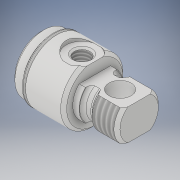
# Autodesk Inventor part: 02P0Y000_rear_head
Saved by Autodesk Inventor 2019 (Build 230136000, 136)
## iProperties
Created: 2023-02-02
Part Number: 02P0Y000_rear_head
Material: Generic
Catalog Web Link: www.cadenas.de
Description: Rear Head-Original Line - Standard Air Cylinders
Vendor: BIMBA
Document SubType Name: Modeling
Designer: psAdmin
Manufacturer: BIMBA
Mass: 2.8315 g
Surface Area: 17.5536 cm^2
Volume: 2.8315 cm^3
Density: 1 g/cm^3
Appearance: PSOLRGB-211-211-211
Category: PARTsolutions
Company: BIMBA
Title: 02P0Y000_rear_head
Author: Cadenas PARTsolutions
Comments: Original Line - Standard Air Cylinders
PSOL_IDENT_0: {$CADENAS_DATA/23d-libs/bimba/bimba_brand/bimba_imperial/bimba_full_line/original_line_cylinders/sta
PSOL_IDENT_1: ndard_air_cylinders/rear_head.prj},241 {VTYP=3D},{NB=02P0Y000_rear_head},{LINA=02P0Y000_rear_head},{
PSOL_IDENT_2: NN=Rear Head},{DATE=26.01.2023 11:43:55},{GEOMDATE=25.01.2022 07:32:02},{VERSION=},{LINEID=30},{WBVA
PSOL_IDENT_3: R=MNT,ACTING,DER,Q,T1,T2,T3,T4,TRIM,Y,K,MB,CUSH,FBON},{WBNUMERIC=TRIM,MB,CUSH}  {NB=02P0Y000_rear_he
PSOL_IDENT_4: ad},{LINA=02P0Y000_rear_head},{KT=DUMMY},{PN=02P0Y000},{BORE=0.56250},{BOREPN=02},{MNT=P},{MNTALG=''
PSOL_IDENT_5: , 'Front Nose' , 'P' , 'Rear Pivot' , 'DX' , 'Double End'},{ACTING=},{ACTINGALG= '' , 'Single Actin
PSOL_IDENT_6: g' },{DER=},{DERALG= '' , 'Standard' },{Q=},{T1=},{T2=},{T3=},{T4=},{TRIM=0},{Y=Y},{K=},{KALG= '', '
PSOL_IDENT_7: without K', 'K', 'with K' },{MB=0},{A1=0.9690},{A1N=0.5000},{A1P=0.9690},{A1B=0.0000},{A1S=0.0000},{
PSOL_IDENT_8: A2=0.157},{A2N=0.1570},{A3=0.0250},{D1=0.6150},{D1N=0.6095},{D1P=0.6150},{D1B=0.0000},{D2=0.5725},{C
PSOL_IDENT_9: 1=0.0300},{C2=0.0300},{NDM=0.1900},{TAB=UNF},{NDMDP=0.2000},{D3=0.1600},{A4=0.1830},{A5=0.4950},{D4=
PSOL_IDENT_10: 0.0000},{A6=0.0000},{A7=0.3750},{A8=0.0000},{D5=0.0000},{D6=0.1540},{A9=0.4400},{NDM2=0.4375},{TAB2=
PSOL_IDENT_11: UNF},{C11=0.0300},{C22=0.0000},{C33=0.0300},{C44=0.0300},{A10=0.3070},{A11=0.0000},{NDM3=0.1900},{ND
PSOL_IDENT_12: M3N=0.1900},{NDM3B=0.0000},{TAB3=UNF},{TAB3N=UNF},{TAB3B=-},{A12=0.406},{A12N=0.4060},{A12B=0.0000},
PSOL_IDENT_13: {A13=0.7810},{D7=0.1570},{D8=0.4355},{A14=0.0620},{A15=0.0775},{D9=0.3600},{R1=0.0315},{X1=0.0000},{
PSOL_IDENT_14: X2=0.0000},{CX=0.0000},{CC=0.0000},{CON=1},{S1=0.0000},{DB=0.0000},{X1B=0.0000},{X2B=0.0000},{A8B=0.
PSOL_IDENT_15: 0000},{A9B=0.0000},{MODEL=1},{NDM4=0.0000},{TAB4=-},{NDM4DP=0.0000},{BC=0.0000},{B1=0.0000},{B2=0.00
PSOL_IDENT_16: 00},{B3=0.0000},{ON=0},{ON2=1},{G1=0.0000},{G2=0.0000},{G3=0.0000},{G4=0.0000},{GD=0.0000},{G5=0.000
PSOL_IDENT_17: 0},{G6=0.0000},{RON=0},{H1=0.0000},{H2=0.0000},{H3=0.0000},{H4=0.0000},{H5=0.0000},{H6=0.0000},{F=0.
PSOL_IDENT_18: 0000},{PNUT=0.5940},{CUSH=0},{CC11=0.000},{CC111=0.0000},{CC22=0.0000},{CC33=0.0000},{CC44=0.0000},{
PSOL_IDENT_19: CC55=0.0000},{CD1=0.0000},{CD2=0.0000},{CD3=0.0000},{CNDM3=0.0000},{CTAB3=0.0000},{OLEN=0.7810},{OD=
PSOL_IDENT_20: 0.2185},{STDIS=0.6250},{STDIS1=0.1560},{BUSHCON=D-8597},{BUSHL=0.3120},{FBON=0},{LCD=0.0000}
NB: 02P0Y000_rear_head
NN: Rear Head
NT: Original Line - Standard Air Cylinders
NBSYN: $PN._rear_head
LINA: 02P0Y000_rear_head
CATALOG: Bimba Products
PN: 02P0Y000
BORE: 0.5625
BOREPN: 02
MNT: Rear Pivot
MNTALG: '' , 'Front Nose' , 'P' , 'Rear Pivot' , 'DX' , 'Double End'
ACTING: Single Acting
DER: Standard
Q: Without Side Ported Rear Head
T1: without T1
T2: without T2
T3: without T3
T4: without T4
TRIM: 0
Y: with Pivot Bushing
K: without K
MB: 0
A1N: 0.5
A1P: 0.969
A1B: 0
A1S: 0
A2N: 0.157
A3: 0.025
D1N: 0.6095
D1P: 0.615
D1B: 0
D2: 0.5725
C1: 0.03
C2: 0.03
TAB: UNF
NDMDP: 0.2
D3: 0.16
A4: 0.183
A5: 0.495
D4: 0
A6: 0
A7: 0.375
A8: 0
D5: 0
D6: 0.154
A9: 0.44
NDM2: 0.4375
TAB2: UNF
C11: 0.03
C22: 0
C33: 0.03
C44: 0.03
A10: 0.307
A11: 0
NDM3N: 0.19
NDM3B: 0
TAB3N: UNF
TAB3B: -
A12N: 0.406
A12B: 0
A13: 0.781
D7: 0.157
D8: 0.4355
A14: 0.062
A15: 0.0775
D9: 0.36
R1: 0.0315
X1: 0
X2: 0
CX: 0
CC: 0
S1: 0
DB: 0
X1B: 0
X2B: 0
A8B: 0
A9B: 0
NDM4: 0
TAB4: -
NDM4DP: 0
BC: 0
B1: 0
B2: 0
B3: 0
G1: 0
G2: 0
G3: 0
G4: 0
GD: 0
G5: 0
G6: 0
H2: 0
H3: 0
F: 0
CUSH: 0
CC111: 0
CC22: 0
CC33: 0
CC44: 0
CC55: 0
CD1: 0
CD2: 0
CD3: 0
CNDM3: 0
CTAB3: 0.0000
OD: 0.2185
STDIS1: 0.156
BUSHCON: D-8597
BUSHL: 0.312
FBON: 0
LCD: 0
SUPPLIER: BIMBA
ARTICLENO: 02P0Y000_rear_head
BOMINFO: 02P0Y000_rear_head
CREATOR: CADENAS GmbH
Autodesk Inventor part; units mm, degrees
sketch "Sketch_18" plane through (0, 0, 0) normal (0, 0, 1) x (1, 0, 0)
  line L0 (13.5128, 0) -> (0, 0)
  line L1 (0, 0) -> (0, 6.5088)
  line L2 (0, 6.5088) -> (0.762, 7.2708)
  line L3 (0.762, 7.2708) -> (2.7178, 7.2708)
  line L4 (2.7178, 7.2708) -> (3.3528, 6.6357)
  line L5 (3.3528, 6.6357) -> (3.9878, 6.6357)
  line L6 (3.9878, 6.6357) -> (3.9878, 7.8105)
  line L7 (3.9878, 7.8105) -> (12.7508, 7.8105)
  line L8 (12.7508, 7.8105) -> (13.5128, 7.0485)
  line L9 (13.5128, 7.0485) -> (13.5128, 0)
  line L10 (13.5128, 0) -> (0, 0)
  constraints: 22 end point
revolve "Revolution1" add sketch "Sketch_18" angle 360 about axis through (13.5128, 0, 0) along (1, 0, 0)
sketch "Sketch_15" plane through (0, 0, 0) normal (0, 0, 1) x (1, 0, 0)
  line L0 (24.6126, 0) -> (13.5128, 0)
  line L1 (13.5128, 0) -> (13.5128, 5.5309)
  line L2 (13.5128, 5.5309) -> (15.0876, 5.5309)
  line L3 (15.0876, 5.5309) -> (15.0876, 5.3721)
  arc A0 (15.0876, 5.3721) -> (15.8877, 4.572) centre (15.8877, 5.3721) ccw
  line L4 (15.8877, 4.572) -> (17.0561, 4.572)
  arc A1 (17.0561, 4.572) -> (17.559, 4.7498) centre (17.0561, 5.3721) ccw
  line L5 (17.559, 4.7498) -> (17.6219, 4.8006)
  line L6 (17.6219, 4.8006) -> (18.3775, 5.5563)
  line L7 (18.3775, 5.5563) -> (23.857, 5.5563)
  line L8 (23.857, 5.5563) -> (24.6126, 4.8006)
  line L9 (24.6126, 4.8006) -> (24.6126, 0)
  line L10 (24.6126, 0) -> (13.5128, 0)
  constraints: 22 end point, 4 point on circle, 2 centre point
revolve "Revolution2" add sketch "Sketch_15" angle 360 about axis through (24.6126, 0, 0) along (1, 0, 0)
thread "Thread1" size "7/16-20 UNF" class "2A" standard "ANSI Unified Screw Threads" full length
sketch "Sketch_70" plane through (24.6126, 0, 0) normal (1, 0, 0) x (0, 0, -1)
  line L0 (-31.242, -15.621) -> (31.242, -15.621)
  line L1 (31.242, -15.621) -> (31.242, 15.621)
  line L2 (31.242, 15.621) -> (-31.242, 15.621)
  line L3 (-31.242, 15.621) -> (-31.242, -15.621)
  line L4 (-15.621, -3.8989) -> (15.621, -3.8989)
  line L5 (15.621, -3.8989) -> (15.621, 3.8989)
  line L6 (15.621, 3.8989) -> (-15.621, 3.8989)
  line L7 (-15.621, 3.8989) -> (-15.621, -3.8989)
  constraints: 16 end point
extrude "Extrusion1" cut sketch "Sketch_70" against normal blind 11.0998
sketch "Sketch4" plane through (0, 0, 0) normal (-1, 0, 0) x (0, 0, 1)
  point P0 (0, 0)
hole "Hole1" at (0, 0, 0) direction (1, 0, 0) diameter 3.9116 depth 12.2936 tip angle 120
sketch "Sketch_45" plane through (0, 0, 0) normal (0, 0, 1) x (1, 0, 0)
  line L0 (10.3124, 6.7945) -> (10.3124, 7.8105)
  line L1 (10.3124, 7.8105) -> (14.2748, 7.8105)
  line L2 (14.2748, 7.8105) -> (14.2748, 6.7945)
  line L3 (14.2748, 6.7945) -> (10.3124, 6.7945)
  line L4 (10.3124, 6.7945) -> (10.3124, 7.8105)
  constraints: 10 end point
revolve "Revolution3" cut sketch "Sketch_45" angle 360 about axis through (10.3124, 6.7945, 0) along (0, -1, 0)
sketch "Sketch_46" plane through (0, 0, 0) normal (0, 0, 1) x (1, 0, 0)
  line L0 (10.3124, 0) -> (10.3124, 8.0645)
  line L1 (10.3124, 8.0645) -> (12.7254, 8.0645)
  line L2 (12.7254, 8.0645) -> (12.7254, 6.7945)
  line L3 (12.7254, 6.7945) -> (12.2961, 6.3652)
  line L4 (12.2961, 6.3652) -> (12.2961, 0)
  line L5 (12.2961, 0) -> (10.3124, 0)
  line L6 (10.3124, 0) -> (10.3124, 8.0645)
  constraints: 14 end point
revolve "Revolution4" cut sketch "Sketch_46" angle 360 about axis through (10.3124, 0, 0) along (0, -1, 0)
thread "Thread2" size "10-32 UNF" class "2B" standard "ANSI Unified Screw Threads" length 4.4094
sketch "Sketch_24" plane through (0, 0, 0) normal (0, 0, 1) x (1, 0, 0)
  line L0 (3.9878, 0) -> (3.3528, 0)
  line L1 (3.1602, 7.8105) -> (3.1602, 7.7263)
  line L2 (3.1602, 7.7263) -> (3.8708, 7.0158)
  arc A0 (3.8708, 6.8362) -> (3.8708, 7.0158) centre (3.781, 6.926) ccw
  line L3 (3.8708, 6.8362) -> (3.6703, 6.6357)
  line L4 (3.6703, 6.6357) -> (3.3528, 6.6357)
  line L5 (3.3528, 6.6357) -> (3.3528, 6.3817)
  line L6 (3.3528, 6.3817) -> (3.9878, 6.3817)
  line L7 (3.9878, 6.3817) -> (3.9878, 7.1861)
  line L8 (3.9878, 7.1861) -> (3.3634, 7.8105)
  line L9 (3.3634, 7.8105) -> (3.1602, 7.8105)
  constraints: 20 end point, 2 point on circle, 1 centre point
revolve "Revolution5" add sketch "Sketch_24" angle 360 about axis through (3.9878, 0, 0) along (1, 0, 0)
sketch "Sketch_43" plane through (0, 0, 0) normal (0, 1, 0) x (-1, 0, 0)
  circle A0 centre (-19.8374, 0) radius 2.775
  constraints: 1 centre point
extrude "Extrusion2" cut sketch "Sketch_43" along normal mid plane 11.6967
ref_plane "1_XY" through (15.0876, 0, 0) normal (1, 0, 0) x (0, 0, -1)
ref_plane "1_YZ" through (15.0876, 0, 0) normal (0, 0, -1) x (0, 1, 0)
ref_plane "1_ZX" through (15.0876, 0, 0) normal (0, 1, 0) x (1, 0, 0)
ref_plane "c1_XY" through (13.5128, 5.5309, 0) normal (0, 0, 1) x (1, 0, 0)
ref_plane "c1_YZ" through (13.5128, 5.5309, 0) normal (1, 0, 0) x (0, 1, 0)
ref_plane "c1_ZX" through (13.5128, 5.5309, 0) normal (0, 1, 0) x (0, 0, 1)
ref_plane "c2_XY" through (13.5128, -5.5309, 0) normal (0, 0, 1) x (1, 0, 0)
ref_plane "c2_YZ" through (13.5128, -5.5309, 0) normal (1, 0, 0) x (0, 1, 0)
ref_plane "c2_ZX" through (13.5128, -5.5309, 0) normal (0, 1, 0) x (0, 0, 1)
ref_plane "cc1_XY" through (13.5128, 0, 0) normal (0, 0, 1) x (1, 0, 0)
ref_plane "cc1_YZ" through (13.5128, 0, 0) normal (1, 0, 0) x (0, 1, 0)
ref_plane "cc1_ZX" through (13.5128, 0, 0) normal (0, 1, 0) x (0, 0, 1)
ref_plane "cc2_XY" through (15.0876, 0, 0) normal (0, 0, 1) x (1, 0, 0)
ref_plane "cc2_YZ" through (15.0876, 0, 0) normal (1, 0, 0) x (0, 1, 0)
ref_plane "cc2_ZX" through (15.0876, 0, 0) normal (0, 1, 0) x (0, 0, 1)
ref_plane "lovra1_XY" through (19.9644, 0, 0) normal (1, 0, 0) x (0, 0, -1)
ref_plane "lovra1_YZ" through (19.9644, 0, 0) normal (0, 0, -1) x (0, 1, 0)
ref_plane "lovra1_ZX" through (19.9644, 0, 0) normal (0, 1, 0) x (1, 0, 0)
ref_plane "lovra2_XY" through (19.9644, 6.2865, 0) normal (1, 0, 0) x (0, 0, -1)
ref_plane "lovra2_YZ" through (19.9644, 6.2865, 0) normal (0, 0, -1) x (0, 1, 0)
ref_plane "lovra2_ZX" through (19.9644, 6.2865, 0) normal (0, 1, 0) x (1, 0, 0)
ref_plane "lovra21_XY" through (0, 0, 5.2705) normal (1, 0, 0) x (0, 0, -1)
ref_plane "lovra21_YZ" through (0, 0, 5.2705) normal (0, 0, -1) x (0, 1, 0)
ref_plane "lovra21_ZX" through (0, 0, 5.2705) normal (0, 1, 0) x (1, 0, 0)
ref_plane "lovra22_XY" through (0, 0, -5.2705) normal (1, 0, 0) x (0, 0, -1)
ref_plane "lovra22_YZ" through (0, 0, -5.2705) normal (0, 0, -1) x (0, 1, 0)
ref_plane "lovra22_ZX" through (0, 0, -5.2705) normal (0, 1, 0) x (1, 0, 0)
ref_plane "lovra3_XY" through (19.9644, -6.2865, 0) normal (1, 0, 0) x (0, 0, -1)
ref_plane "lovra3_YZ" through (19.9644, -6.2865, 0) normal (0, 0, -1) x (0, 1, 0)
ref_plane "lovra3_ZX" through (19.9644, -6.2865, 0) normal (0, 1, 0) x (1, 0, 0)
ref_plane "olen_XY" through (19.8374, 0, 0) normal (1, 0, 0) x (0, 0, -1)
ref_plane "olen_YZ" through (19.8374, 0, 0) normal (0, 0, -1) x (0, 1, 0)
ref_plane "olen_ZX" through (19.8374, 0, 0) normal (0, 1, 0) x (1, 0, 0)
ref_plane "p1_XY" through (24.6126, 0, 3.9624) normal (1, 0, 0) x (0, 0, -1)
ref_plane "p1_YZ" through (24.6126, 0, 3.9624) normal (0, 0, -1) x (0, 1, 0)
ref_plane "p1_ZX" through (24.6126, 0, 3.9624) normal (0, 1, 0) x (1, 0, 0)
ref_plane "p2_XY" through (24.6126, 0, -3.9624) normal (1, 0, 0) x (0, 0, -1)
ref_plane "p2_YZ" through (24.6126, 0, -3.9624) normal (0, 0, -1) x (0, 1, 0)
ref_plane "p2_ZX" through (24.6126, 0, -3.9624) normal (0, 1, 0) x (1, 0, 0)
ref_plane "port_XY" through (10.3124, 0, 0) normal (0, 0, 1) x (1, 0, 0)
ref_plane "port_YZ" through (10.3124, 0, 0) normal (1, 0, 0) x (0, 1, 0)
ref_plane "port_ZX" through (10.3124, 0, 0) normal (0, 1, 0) x (0, 0, 1)
ref_plane "port2_XY" through (24.6126, 0, 0) normal (1, 0, 0) x (0, 0, -1)
ref_plane "port2_YZ" through (24.6126, 0, 0) normal (0, 0, -1) x (0, 1, 0)
ref_plane "port2_ZX" through (24.6126, 0, 0) normal (0, 1, 0) x (1, 0, 0)
ref_plane "thd1_XY" through (24.6126, 0, 5.5563) normal (1, 0, 0) x (0, 0, -1)
ref_plane "thd1_YZ" through (24.6126, 0, 5.5563) normal (0, 0, -1) x (0, 1, 0)
ref_plane "thd1_ZX" through (24.6126, 0, 5.5563) normal (0, 1, 0) x (1, 0, 0)
ref_plane "thd2_XY" through (24.6126, 0, -5.5563) normal (1, 0, 0) x (0, 0, -1)
ref_plane "thd2_YZ" through (24.6126, 0, -5.5563) normal (0, 0, -1) x (0, 1, 0)
ref_plane "thd2_ZX" through (24.6126, 0, -5.5563) normal (0, 1, 0) x (1, 0, 0)
ref_plane "to_mounting_bracket_XY" through (13.5128, 0, 0) normal (1, 0, 0) x (0, 0, -1)
ref_plane "to_mounting_bracket_YZ" through (13.5128, 0, 0) normal (0, 0, -1) x (0, 1, 0)
ref_plane "to_mounting_bracket_ZX" through (13.5128, 0, 0) normal (0, 1, 0) x (1, 0, 0)
ref_plane "to_nut_XY" through (15.0876, 0, 0) normal (1, 0, 0) x (0, 0, -1)
ref_plane "to_nut_YZ" through (15.0876, 0, 0) normal (0, 0, -1) x (0, 1, 0)
ref_plane "to_nut_ZX" through (15.0876, 0, 0) normal (0, 1, 0) x (1, 0, 0)
ref_plane "to_pin_XY" through (19.8374, 0, 0) normal (0, 1, 0) x (1, 0, 0)
ref_plane "to_pin_YZ" through (19.8374, 0, 0) normal (1, 0, 0) x (0, 0, -1)
ref_plane "to_pin_ZX" through (19.8374, 0, 0) normal (0, 0, -1) x (0, 1, 0)
ref_plane "to_pin_1_XY" through (19.8374, 0, 0) normal (0, 0, 1) x (1, 0, 0)
ref_plane "to_pin_1_YZ" through (19.8374, 0, 0) normal (1, 0, 0) x (0, 1, 0)
ref_plane "to_pin_1_ZX" through (19.8374, 0, 0) normal (0, 1, 0) x (0, 0, 1)
ref_plane "to_pin_r_XY" through (19.8374, 0, 0) normal (0, 0, 1) x (1, 0, 0)
ref_plane "to_pin_r_YZ" through (19.8374, 0, 0) normal (1, 0, 0) x (0, 1, 0)
ref_plane "to_pin_r_ZX" through (19.8374, 0, 0) normal (0, 1, 0) x (0, 0, 1)
ref_plane "to_screw_XY" through (10.3124, 0, 0) normal (0, 1, 0) x (1, 0, 0)
ref_plane "to_screw_YZ" through (10.3124, 0, 0) normal (1, 0, 0) x (0, 0, -1)
ref_plane "to_screw_ZX" through (10.3124, 0, 0) normal (0, 0, -1) x (0, 1, 0)
ref_plane "to_tube_XY" through (3.3528, 0, 0) normal (1, 0, 0) x (0, 0, -1)
ref_plane "to_tube_YZ" through (3.3528, 0, 0) normal (0, 0, -1) x (0, 1, 0)
ref_plane "to_tube_ZX" through (3.3528, 0, 0) normal (0, 1, 0) x (1, 0, 0)
body "Solid1"
